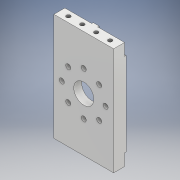
# Autodesk Inventor part: new_base_u106_long_newbearing
Saved by Autodesk Inventor 2018 (Build 220112000, 112)
## iProperties
Created: 2016-12-19
Part Number: new_base_u106_long_newbearing
Material: Aluminum 2014-T4
Document SubType Name: Modeling
Designer: steve
Density: 2.8 g/cm^3
Appearance: Satin
Mass: 19.1708 g
Surface Area: 51.0556 cm^2
Volume: 6.8467 cm^3
Vendor: Rhoban
Author: steve
Autodesk Inventor part; units mm, degrees
ref_plane "YZ Plane" through (0, 0, 0) normal (1, 0, 0) x (0, 1, 0)
ref_plane "XZ Plane" through (0, 0, 0) normal (0, 1, 0) x (-1, 0, 0)
ref_plane "XY Plane" through (0, 0, 0) normal (0, 0, 1) x (1, 0, 0)
sketch "Sketch1" plane through (0, 0, 0) normal (0, 1, 0) x (-1, 0, 0)
  line L0 (15, 27) -> (-15, 27)
  line L1 (-15, 27) -> (-15, -27)
  line L2 (-15, -27) -> (15, -27)
  line L3 (15, -27) -> (15, 27)
  line L4 (0, 27) -> (0, -27) construction
  line L5 (15, 0) -> (-15, 0) construction
  point P0 (0, 0)
  point P1 (0, 0)
  point P2 (15, 0)
  dimension "d0" = 54
  dimension "d1" = 30
  constraints: 12 end point, 6 midpoint, 2 parallel, 2 perpendicular, 1 coincident, 1 horizontal, 1 point on line
  measures "d0" distance of L2.end L0.start
  measures "d1" distance between parallel lines of L1 L3
extrude "Extrusion1" add sketch "Sketch1" along normal blind 6.25
sketch "Sketch2" plane through (0, 6.25, 0) normal (0, 1, 0) x (1, 0, 0)
  circle A0 centre (0, 0) radius 11 construction
  line L0 (0, 0) -> (-15, 0) construction
  line L1 (-35.2782, 0) -> (23.3797, 0) construction
  line L2 (0, 37.8) -> (0, -37.8) construction
  line L3 (-15, -27) -> (15, -27) projected
  line L4 (15, -27) -> (15, 27) projected
  line L5 (15, 27) -> (-15, 27) projected
  line L6 (-15, 27) -> (-15, -27) projected
  line L7 (-15, 27) -> (-15, -27) projected
  point P0 (-11, 0)
  point P1 (-7.7782, -7.7782)
  point P2 (0, -11)
  point P3 (7.7782, -7.7782)
  point P4 (11, 0)
  point P5 (7.7782, 7.7782)
  point P6 (0, 11)
  point P7 (-7.7782, 7.7782)
  dimension "d7" = 22
  dimension "d8" = 360
  constraints: 2 end point, 1 coincident, 1 collinear, 1 horizontal alignment, 1 midpoint, 1 point on line, 11 other
hole "Hole1" at (-11, 6.25, 0) at (-7.7782, 6.25, -7.7782) at (0, 6.25, -11) at (7.7782, 6.25, -7.7782) at (11, 6.25, 0) at (7.7782, 6.25, 7.7782) at (0, 6.25, 11) at (-7.7782, 6.25, 7.7782) direction (0, -1, 0) diameter 2.5 end through all
sketch "Sketch3" plane through (0, 6.25, 0) normal (0, 1, 0) x (1, 0, 0)
  circle A0 centre (0, 0) radius 5.05
  dimension "d17" = 10.1
  constraints: 1 centre point, 1 coincident
  measures "d17" diameter of A0
extrude "Extrusion2" cut sketch "Sketch3" against normal through all
sketch "Sketch6" plane through (-15, 0, 27) normal (0, 0, 1) x (1, 0, 0)
  line L0 (-10.3797, 2.75) -> (37.9037, 2.75) construction
  line L1 (0, 0) -> (30, 0) construction
  line L2 (0, 0) -> (0, 6.25) projected
  point P0 (15, 0)
  point P1 (4.5, 2.75)
  point P2 (11.5, 2.75)
  point P3 (18.5, 2.75)
  point P4 (25.5, 2.75)
  dimension "d33" = 2.75
  dimension "d34" = 4.5
  dimension "d37" = 7
  constraints: 2 end point, 2 horizontal, 1 point on line, 3 other
  measures "d33" distance between parallel lines of L1 L0
  measures "d34" distance from line of L2 point (4.5, 2.75)
  measures "d37" distance of point (4.5, 2.75) point (11.5, 2.75)
hole "Hole3" at (-10.5, 2.75, 27) at (-3.5, 2.75, 27) at (3.5, 2.75, 27) at (10.5, 2.75, 27) direction (0, 0, -1) diameter 2.013 depth 7.6 tip angle 118 thread size "M2.5x0.45" class "6H" standard "ANSI Metric M Profile"
sketch "Sketch7" plane through (15, 0, -27) normal (0, 0, -1) x (-1, 0, 0)
  line L0 (-10.51, 2.75) -> (37.7733, 2.75) construction
  line L1 (0, 0) -> (29.8697, 0) construction
  line L2 (0, 0) -> (0, 3.7534)
  line L3 (0, 0) -> (30, 0) projected
  line L4 (0, 0) -> (0, 6.25) projected
  point P0 (15, 0)
  point P1 (15, 0)
  point P2 (4.5, 2.75)
  point P3 (11.5, 2.75)
  point P4 (18.5, 2.75)
  point P5 (25.5, 2.75)
  dimension "d53" = 2.75
  dimension "d54" = 4.5
  dimension "d55" = 7
  constraints: 6 end point, 2 collinear, 2 horizontal, 1 point on line, 3 other
  measures "d53" distance between parallel lines of L1 L0
  measures "d54" distance from line of L2 point (4.5, 2.75)
  measures "d55" distance of point (4.5, 2.75) point (11.5, 2.75)
hole "Hole4" at (10.5, 2.75, -27) at (-10.5, 2.75, -27) at (-3.5, 2.75, -27) at (3.5, 2.75, -27) direction (0, 0, 1) diameter 2.013 depth 7.6 tip angle 118 thread size "M2.5x0.45" class "6H" standard "ANSI Metric M Profile"
sketch "Sketch8" plane through (0, 6.25, 0) normal (0, 1, 0) x (1, 0, 0)
  line L0 (0, 38.85) -> (0, -39.55) construction
  line L1 (-15, -27) -> (15, -27) projected
  line L2 (15, 27) -> (-15, 27) projected
  line L3 (-1.5, -27) -> (-15, -27)
  line L4 (-15, -27) -> (-15, -21)
  line L5 (-15, -21) -> (-1.5, -21)
  line L6 (1.5, -27) -> (15, -27)
  line L7 (15, -27) -> (15, -21)
  line L8 (15, -21) -> (1.5, -21)
  line L9 (15, -27) -> (15, 27) projected
  line L10 (-15, 27) -> (-15, -27) projected
  line L11 (-1.5, -21) -> (-1.5, -27)
  line L12 (-15, -27) -> (15, -27) projected
  line L13 (1.5, -21) -> (1.5, -27)
  line L14 (-15, 0) -> (15, 0) construction
  line L15 (-1.5, 27) -> (-15, 27)
  line L16 (-15, 27) -> (-15, 21)
  line L17 (-15, 21) -> (-1.5, 21)
  line L18 (1.5, 27) -> (15, 27)
  line L19 (15, 27) -> (15, 21)
  line L20 (15, 21) -> (1.5, 21)
  line L21 (-1.5, 21) -> (-1.5, 27)
  line L22 (1.5, 21) -> (1.5, 27)
  line L23 (-21.8515, -25) -> (23.2072, -25) construction
  point P0 (0, 0)
  dimension "d80" = 6
  dimension "d81" = 3
  dimension "d82" = 13.5
  dimension "d86" = 2
  constraints: 36 end point, 7 symmetric about line, 4 point on line, 3 collinear, 3 horizontal, 3 parallel, 3 perpendicular, 2 midpoint
  measures "d80" distance between parallel lines of L1 L5
  measures "d81" distance between parallel lines of L13 L11
  measures "d82" distance between parallel lines of L7 L13
  measures "d86" distance between parallel lines of L1 L23
extrude "Extrusion6" cut sketch "Sketch8" against normal blind 0.75 contours L4 L5 L11 L1 | L13 L8 L7 L1 | L10 L2 L21 L17 | L20 L22 L2 L9
fillet "Fillet1" radius 3 4 edges at (1.5, 5.875, 21) (-1.5, 5.875, 21) (1.5, 5.875, -21) (-1.5, 5.875, -21)
sketch "Sketch11" plane through (0, 6.25, 0) normal (0, 1, 0) x (1, 0, 0)
  line L0 (-13.5, -19.5) -> (13.5, -19.5)
  line L1 (13.5, -19.5) -> (13.5, 19.5)
  line L2 (13.5, 19.5) -> (-13.5, 19.5)
  line L3 (-13.5, 19.5) -> (-13.5, -19.5)
  line L4 (-15, 21) -> (-15, -21) projected
  line L5 (15, -21) -> (15, 21) projected
  line L6 (-1.5, -27) -> (-15, -27) projected
  line L7 (-15, 27) -> (-1.5, 27) projected
  point P0 (0, 0)
  dimension "d87" = 7.5
  dimension "d88" = 7.5
  dimension "d91" = 1.5
  dimension "d92" = 1.5
  constraints: 8 end point, 2 parallel, 1 horizontal, 1 perpendicular
  measures "d87" distance between parallel lines of L6 L0
  measures "d88" distance between parallel lines of L7 L2
  measures "d91" distance between parallel lines of L4 L3
  measures "d92" distance between parallel lines of L5 L1
extrude "Extrusion7" cut sketch "Sketch11" against normal blind 2.25
fillet "Fillet2" radius 1.5 4 edges at (-13.5, 5.125, 19.5) (13.5, 5.125, 19.5) (13.5, 5.125, -19.5) (-13.5, 5.125, -19.5)
equation "\"d0\" = u_internal_width + 2 * u_side_trace_depth"
equation "\"d1\" = u_internal_depth"
equation "\"d3\" = plate_thickness"
equation "\"d7\" = d9"
equation "\"d18\" = plate_thickness"
equation "\"d33\" = hole_2_bottom"
equation "\"d53\" = hole_2_bottom"
equation "\"d83\" = plate_thickness - border_thickness"
equation "\"plate_thickness\" = 6.25"
equation "\"d9\" = 22"
equation "\"tol\" = 0.1"
equation "\"u_internal_width\" = 52"
equation "\"u_internal_depth\" = 30"
equation "\"u_side_trace_depth\" = 1"
equation "\"border_thickness\" = 5.5"
equation "\"hole_2_bottom\" = 0.5 * border_thickness"
body "Solid1"
